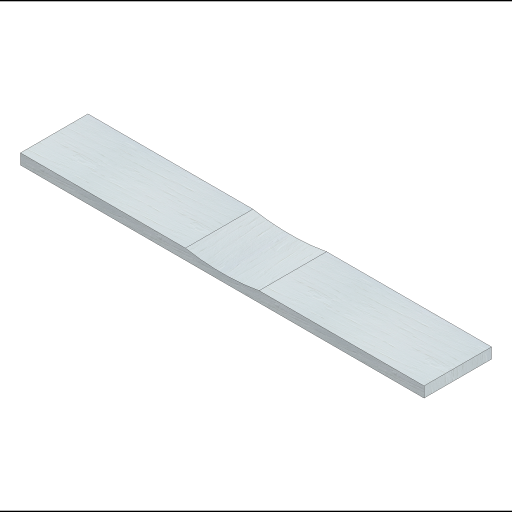
# Autodesk Inventor part: Exhaust Frame Upper+Lower as-built
Saved by Autodesk Inventor 2023 (Build 270158000, 158)
## iProperties
Created: 2022-03-08
Part Number: Exhaust Frame Upper+Lower as-built
Material: Wood (Oak)
Document SubType Name: Modeling
Designer: kamer
Density: 0.76 g/cm^3
Appearance: Wood - Painted White
Author: kamer
Autodesk Inventor part; units mm, degrees
ref_plane "YZ Plane" through (0, 0, 0) normal (1, 0, 0) x (0, 1, 0)
ref_plane "XZ Plane" through (0, 0, 0) normal (0, 1, 0) x (-1, 0, 0)
ref_plane "XY Plane" through (0, 0, 0) normal (0, 0, 1) x (1, 0, 0)
sketch "Sketch1" plane through (0, 0, 0) normal (0, 0, 1) x (1, 0, 0)
  line L0 (0, 0) -> (455.6125, 0)
  line L1 (455.6125, 0) -> (455.6125, 11.938)
  line L2 (455.6125, 11.938) -> (0, 11.938)
  line L3 (0, 11.938) -> (0, 0)
  dimension "d0" = 455.6125
  dimension "d1" = 11.938
  constraints: 8 end point, 2 parallel, 1 horizontal, 1 perpendicular
  measures "d0" distance of L2.end L1.end
  measures "d1" distance of L1.end L0.end
extrude "Extrusion1" add sketch "Sketch1" along normal blind 76.2
sketch "Sketch2" plane through (0, 0, 76.2) normal (0, 0, 1) x (1, 0, 0)
  circle A0 centre (227.8126, 236.728) radius 228.6
  line L0 (455.6125, 11.938) -> (0, 11.938) projected
  line L1 (0, 11.938) -> (0, 0) projected
  dimension "d6" = 227.8126
  dimension "d7" = 224.79
  dimension "d8" = 457.2
  constraints: 1 centre point
  measures "d6" distance from line of L1 A0.centre
  measures "d7" distance from line of L0 A0.centre
  measures "d8" diameter of A0
extrude "Extrusion2" cut sketch "Sketch2" against normal through all
body "Solid1"
